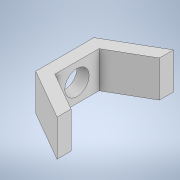
# Autodesk Inventor part: GearboxDogHolder
Saved by Autodesk Inventor 2022 (Build 260153000, 153)
## iProperties
Created: 2022-02-13
Part Number: GearboxDogHolder
Material: Generic
Document SubType Name: Modeling
Designer: merky
Density: 1 g/cm^3
Appearance: Default
Author: merky
Autodesk Inventor part; units mm, degrees
ref_plane "YZ Plane" through (0, 0, 0) normal (1, 0, 0) x (0, 1, 0)
ref_plane "XZ Plane" through (0, 0, 0) normal (0, 1, 0) x (-1, 0, 0)
ref_plane "XY Plane" through (0, 0, 0) normal (0, 0, 1) x (1, 0, 0)
sketch "Sketch1" plane through (0, 0, 0) normal (0, 1, 0) x (-1, 0, 0)
  line L0 (0, 9.2388) -> (8.001, 4.6194)
  line L1 (8.001, 4.6194) -> (8.001, -4.6194)
  line L2 (8.001, -4.6194) -> (0, -9.2388)
  line L3 (10.541, -6.0858) -> (0, -12.1717)
  line L4 (0, 12.1717) -> (10.541, 6.0858)
  line L5 (10.541, 6.0858) -> (10.541, -6.0858)
  line L6 (0, 12.1717) -> (0, 9.2388)
  line L7 (0, -9.2388) -> (0, -12.1717)
  point P0 (0, 0)
  point P1 (0, 0)
  point P2 (0, 0)
  point P3 (0, 0)
  dimension "d5" = 2.54
  constraints: 16 end point, 3 coincident, 1 collinear, 1 vertical, 12 other
  measures "d5" distance between parallel lines of L5 L1
extrude "Extrusion1" add sketch "Sketch1" along normal blind 7.62
sketch "Sketch2" plane through (-10.541, 0, -6.0858) normal (-1, 0, 0) x (0, 0, 1)
  circle A0 centre (6.0833, 3.81) radius 2.54
  line L0 (0, 0) -> (12.1717, 0) projected
  line L1 (12.1717, 0) -> (12.1717, 7.62) projected
  line L2 (0, 0) -> (0, 7.62) projected
  point P0 (6.0858, 0)
  dimension "d8" = 5.08
  dimension "d9" = 3.81
  dimension "d10" = 12.1717
  dimension "d11" = 6.0833
  constraints: 1 centre point
  measures "d8" diameter of A0
  measures "d9" distance from line of L0 A0.centre
  measures "d10" distance between parallel lines of L1 L2
  measures "d11" distance from line of L2 A0.centre
extrude "Extrusion2" cut sketch "Sketch2" against normal through all
body "Solid1"
